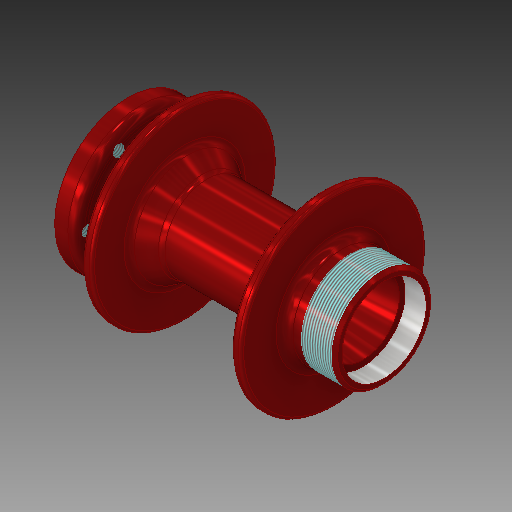
# Autodesk Inventor part: BackWheel
Saved by Autodesk Inventor 2019.2 (Build 232265000, 265)
## iProperties
Created: 2017-11-19
Part Number: BackWheel
Material: Generic
Document SubType Name: Modeling
Designer: eroldan
Density: 1 g/cm^3
Appearance: Default
Author: eroldan
Autodesk Inventor part; units mm, degrees
note: some values were not read from the file. Chosen so that the rebuilt part matches the saved one: direction of "Hole2".
ref_plane "YZ Plane" through (0, 0, 0) normal (1, 0, 0) x (0, 1, 0)
ref_plane "XZ Plane" through (0, 0, 0) normal (0, 1, 0) x (-1, 0, 0)
ref_plane "XY Plane" through (0, 0, 0) normal (0, 0, 1) x (1, 0, 0)
sketch "Sketch2" plane through (0, 0, 0) normal (0, 0, 1) x (1, 0, 0)
  line L0 (95.5, 15) -> (60, 15)
  line L1 (58.65, 10) -> (96.85, 10)
  line L2 (53, 20) -> (53, 33)
  line L3 (53, 33) -> (49.5, 33)
  line L4 (49.5, 19) -> (49.5, 33)
  line L5 (49.5, 19) -> (40.5, 19)
  line L6 (40.5, 19) -> (40.5, 26)
  line L7 (40.5, 26) -> (32.85, 26)
  line L8 (32.85, 26) -> (32.85, 15)
  line L9 (102.5, 20) -> (102.5, 33)
  line L10 (102.5, 33) -> (106, 33)
  line L11 (106, 17.5) -> (106, 33)
  line L12 (32.85, 15) -> (40.35, 15)
  line L13 (116.35, 13) -> (116.35, 15)
  line L14 (116.35, 15) -> (123.85, 15)
  line L15 (123.85, 15) -> (123.85, 17.5)
  line L16 (123.85, 17.5) -> (106, 17.5)
  line L17 (60, 15) -> (53, 20)
  line L18 (102.5, 20) -> (95.5, 15)
  line L19 (9.75, 17.0467) -> (9.75, -22.4939)
  line L20 (145.75, 17.0467) -> (145.75, -22.4939)
  line L21 (-29.15, 0) -> (174.9, 0) construction
  line L22 (40.35, 15) -> (40.35, 13)
  line L23 (40.35, 13) -> (58.65, 10)
  line L24 (116.35, 13) -> (96.85, 10)
  point P0 (0, 0)
  point P1 (102.5, 15)
  point P2 (53, 15)
  point P3 (125.35, 0)
  point P4 (31.85, 0)
  point P5 (77.75, 10)
  point P6 (77.75, 15)
  dimension "d53" = 9
  dimension "d54" = 16.65
  dimension "d77" = 9
  dimension "d78" = 7.5
  dimension "d83" = 5
  dimension "d84" = 7
  dimension "d119" = 56.5
  dimension "d120" = 93.5
  dimension "d121" = 39.75
  dimension "d122" = 17.85
  dimension "d123" = 10
  dimension "d124" = 15
  dimension "d125" = 33
  dimension "d126" = 3.5
  dimension "d127" = 3.5
  dimension "d129" = 5
  dimension "d130" = 7
  dimension "d131" = 5
  dimension "d132" = 19
  dimension "d133" = 17.5
  dimension "d134" = 2
  dimension "d135" = 38.2
  dimension "d137" = 7.5
  dimension "d139" = 2
  dimension "d140" = 26
  dimension "d141" = 136
  constraints: 48 end point, 7 vertical, 6 horizontal, 5 perpendicular, 4 point on line, 2 collinear, 2 midpoint, 1 vertical alignment, 4 other
  measures "d53" distance of L4.start L5.end
  measures "d54" distance between parallel lines of L4 L8
  measures "d77" distance from line of L13 point (125.35, 0)
  measures "d78" distance of L13.end L14.end
  measures "d83" distance of L9.start point (102.5, 15)
  measures "d84" distance of L0.start point (102.5, 15)
  measures "d119" distance between parallel lines of L11 L4
  measures "d120" distance of point (125.35, 0) point (31.85, 0)
  measures "d121" distance between parallel lines of L19 L4
  measures "d122" distance of L15.end L11.start
  measures "d123" distance between parallel lines of L21 L1
  measures "d124" distance between parallel lines of L21 L14
  measures "d125" distance between parallel lines of L21 L3
  measures "d126" distance between parallel lines of L11 L9
  measures "d127" distance between parallel lines of L4 L2
  measures "d129" distance of point (53, 15) L2.start
  measures "d130" distance of point (53, 15) L0.end
  measures "d131" distance between parallel lines of L0 L1
  measures "d132" distance between parallel lines of L21 L5
  measures "d133" distance between parallel lines of L21 L16
  measures "d134" distance of L12.end L22.end
  measures "d135" distance of L1.start L1.end
  measures "d137" distance of L8.end L12.end
  measures "d139" distance of L13.start L13.end
  measures "d140" distance between parallel lines of L21 L7
  measures "d141" distance between parallel lines of L19 L20
revolve "Revolution1" add sketch "Sketch2" angle 360 about axis through (-10, 0, 0) along (1, 0, 0)
fillet "Fillet6" radius 3 8 edges at (49.5, -19, 0) (40.5, -19, 0) (40.5, -26, 0) (106, -17.5, 0) (102.5, -20, 0) (95.5, -15, 0) (60, -15, 0) (53, -20, 0)
fillet "Fillet6" radius 1 4 edges at (53, -33, 0) (49.5, -33, 0) (106, -33, 0) (102.5, -33, 0)
thread "Thread1" size "R 1/16" standard "ISO Taper" length 12
chamfer "Chamfer2" distance 1 angle 45 1 edges at (123.85, -17.5, 0)
sketch "Sketch6" plane through (32.85, 0, 0) normal (-1, 0, 0) x (0, 0, 1)
  point P0 (0, 0)
  point P1 (22, 0)
  dimension "d94" = 22
  measures "d94" distance of point (22, 0) point (0, 0)
hole "Hole2" at (32.85, 0, 22) direction (1, 0, 0) diameter 4.134 end up to surface thread size "M5x0.8" class "6H" standard "ISO Metric profile"
pattern_circular "Circular Pattern2" count 6 over 360 about axis through (-10, 0, 0) along (1, 0, 0) of "Hole2"
body "Solid1"
